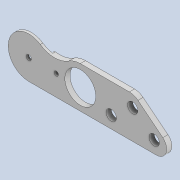
# Autodesk Inventor part: 揺動節左
Saved by Autodesk Inventor 2020.4 (Build 244396000, 396)
## iProperties
Created: 2021-05-01
Part Number: 揺動節左
Material: 一般
Document SubType Name: Modeling
Designer: happy
Density: 1 g/cm^3
Appearance: 既定
Mass: 5.63365 g
Surface Area: 51.3056 cm^2
Volume: 5.63365 cm^3
Author: happy
Autodesk Inventor part; units mm, degrees
ref_plane "YZ Plane" through (0, 0, 0) normal (1, 0, 0) x (0, 1, 0)
ref_plane "XZ Plane" through (0, 0, 0) normal (0, 1, 0) x (-1, 0, 0)
ref_plane "XY Plane" through (0, 0, 0) normal (0, 0, 1) x (1, 0, 0)
sketch "スケッチ1" plane through (0, 0, 0) normal (0, 0, 1) x (1, 0, 0)
  line L0 (0, 0) -> (30, 0) construction
  line L1 (0, 12) -> (30.0122, 12)
  line L2 (30, -12) -> (0, -12)
  arc A0 (0, 12) -> (0, -12) centre (0, 0) ccw
  arc A1 (30, -12) -> (30.0122, 12) centre (30, 0) ccw
  circle A2 centre (0, 0) radius 1.5
  circle A3 centre (30, 0) radius 9.025
  arc A4 (6.6694, 9.9759) -> (23.3428, 9.9759) centre (15.0061, 22.4459) ccw
  arc A5 (30.0122, 12) -> (30, -12) centre (30.0122, 0) ccw construction
  arc A6 (0, -12) -> (0, 12) centre (0, 0) ccw construction
  arc A7 (6.6694, 9.9759) -> (0, 12) centre (0, 0) ccw
  arc A8 (30.0122, 12) -> (23.3428, 9.9759) centre (30.0122, 0) ccw
  line L3 (30.0122, 12) -> (92.8308, 12)
  line L4 (92.8308, 12) -> (92.8308, -12)
  line L5 (92.8308, -12) -> (30.0122, -12)
  line L6 (30.0122, -12) -> (30.0122, 12)
  circle A9 centre (16, 0) radius 1.25
  point P0 (30.0122, -12)
  dimension "d0" = 30
  dimension "d1" = 12
  dimension "d2" = 3
  dimension "d3" = 18.05
  dimension "d6" = 15
  dimension "d11" = 2.5
  dimension "d12" = 16
  constraints: 16 end point, 15 point on circle, 10 centre point, 10 tangent, 3 coincident, 3 parallel, 2 concentric, 2 horizontal, 1 perpendicular, 1 point on line
  measures "d0" distance of L0.start L0.end
  measures "d1" radius of A1
  measures "d2" diameter of A2
  measures "d3" diameter of A3
  measures "d6" radius of A4
  measures "d11" diameter of A9
  measures "d12" distance of A2.centre A9.centre
extrude "押し出し1" add sketch "スケッチ1" along normal blind 3 contours A7 A4 A8 L6 A3 A1 L2 A0 | L3 L4 L5 A1 | A1 L6 A3
sketch "スケッチ2" plane through (0, 0, 0) normal (0, 0, -1) x (-1, 0, 0)
  arc A0 (-30.0122, -12) -> (-30, -12) centre (-30, 0) ccw projected
  line L0 (-92.8308, 12) -> (-30.0122, 12) projected
  line L1 (-92.8308, -12) -> (-92.8308, 12) projected
  line L2 (0, -12) -> (-30, -12) projected
  arc A1 (0, -12) -> (-6.6694, 9.9759) centre (0, 0) ccw projected
  arc A2 (-23.3428, 9.9759) -> (-6.6694, 9.9759) centre (-15.0061, 22.4459) ccw projected
  circle A3 centre (0, 0) radius 1.5 projected
  circle A4 centre (-30, 0) radius 9.025 projected
  arc A5 (-23.3428, 9.9759) -> (-6.6694, 9.9759) centre (-15.0061, 22.4459) ccw projected
  arc A6 (-6.6694, 9.9759) -> (0, -12) centre (0, 0) ccw
  arc A7 (-7.8, 10.4) -> (0, -13) centre (0, 0) ccw
  line L3 (-30.0122, -12) -> (-92.8308, -12) projected
  arc A8 (-23.3428, 9.9759) -> (-30.0122, 12) centre (-30.0122, 0) ccw projected
  point P0 (-9.9986, 8.3083)
  point P1 (-5, -12)
  point P2 (-10.0009, 8.3056)
  dimension "d7" = 1
  constraints: 4 point on circle, 2 centre point, 1 concentric, 1 tangent
  measures "d7" radial gap between concentric circles of A6 A7
extrude "押し出し2" cut sketch "スケッチ2" against normal blind 1.5 contours A7 A2 A6 L2 | A6 A1
fillet "フィレット1" radius 1 2 edges at (10.0009, 8.3056, 0.75) (5, -12, 0.75)
sketch "スケッチ3" plane through (0, 0, 3) normal (0, 0, 1) x (1, 0, 0)
  line L0 (92.8308, 12) -> (30.0122, 12) projected
  arc A0 (30.0122, 12) -> (23.3428, 9.9759) centre (30.0122, 0) ccw projected
  arc A1 (6.6694, 9.9759) -> (23.3428, 9.9759) centre (15.0061, 22.4459) ccw projected
  arc A2 (6.6694, 9.9759) -> (0, -12) centre (0, 0) ccw projected
  line L1 (0, -12) -> (30, -12) projected
  arc A3 (30, -12) -> (30.0122, -12) centre (30, 0) ccw projected
  line L2 (30.0122, -12) -> (92.8308, -12) projected
  line L3 (92.8308, -12) -> (92.8308, 12) projected
  circle A4 centre (30, 0) radius 9.025 projected
  circle A5 centre (0, 0) radius 1.5 projected
  circle A6 centre (16, 0) radius 1.25 projected
  circle A7 centre (48, -5) radius 3.025
  circle A8 centre (73, -5) radius 3.025
  circle A9 centre (60.5, 5) radius 3.025
  line L4 (48, -5) -> (73, -5) construction
  line L5 (92.8308, 12) -> (30.0122, 12) projected
  line L6 (61.3547, 12) -> (92.8308, -13.1809)
  line L7 (92.8308, -12) -> (92.8308, 12) projected
  line L8 (60.5, 5) -> (73, -5) construction
  line L9 (60.5, 5) -> (60.5, -5) construction
  point P0 (60.5, 0)
  point P1 (91.3547, -12)
  dimension "d13" = 6.05
  dimension "d14" = 6.05
  dimension "d15" = 6.05
  dimension "d16" = 25
  dimension "d17" = 10
  dimension "d18" = 18
  dimension "d19" = 6
  constraints: 8 end point, 3 centre point, 2 midpoint, 2 point on line, 1 horizontal, 1 horizontal alignment, 1 parallel, 1 vertical, 1 vertical alignment
  measures "d13" diameter of A7
  measures "d14" diameter of A8
  measures "d15" diameter of A9
  measures "d16" distance of L4.end L4.start
  measures "d17" vertical distance of L8.start L4.start
  measures "d18" horizontal distance of A4.centre L4.start
  measures "d19" distance between parallel lines of L6 L8
extrude "押し出し3" cut sketch "スケッチ3" against normal blind 10 contours L3 L2 L6 L0 | A7 | A8 | A9
fillet "フィレット2" radius 8 1 edges at (61.3547, 12, 1.5)
fillet "フィレット3" radius 6 1 edges at (91.3547, -12, 1.5)
